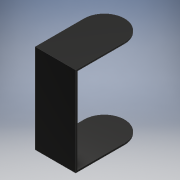
# Autodesk Inventor part: Wrist U-Plate
Saved by Autodesk Inventor 2017 (Build 210142000, 142)
## iProperties
Created: 2018-10-18
Part Number: Wrist U-Plate
Material: Generic
Document SubType Name: Modeling
Designer: Cameron
Density: 1 g/cm^3
Appearance: Glossy - Black
Author: Cameron
Autodesk Inventor part; units mm, degrees
ref_plane "YZ Plane" through (0, 0, 0) normal (1, 0, 0) x (0, 1, 0)
ref_plane "XZ Plane" through (0, 0, 0) normal (0, 1, 0) x (-1, 0, 0)
ref_plane "XY Plane" through (0, 0, 0) normal (0, 0, 1) x (1, 0, 0)
sketch "Sketch1" plane through (0, 0, 0) normal (0, 1, 0) x (-1, 0, 0)
  line L0 (0, 0) -> (24, 0)
  line L1 (24, 0) -> (24, -53)
  line L2 (24, -53) -> (0, -53)
  line L3 (0, -53) -> (0, 0)
  dimension "d0" = 24
  dimension "d1" = 53
  constraints: 8 end point, 2 parallel, 1 horizontal, 1 perpendicular
  measures "d0" distance of L1.end L2.end
  measures "d1" distance of L0.end L1.end
extrude "Extrusion1" add sketch "Sketch1" along normal blind 1
sketch "Sketch2" plane through (0, 1, 0) normal (0, 1, 0) x (1, 0, 0)
  line L0 (-24, 0) -> (0, 0) projected
  line L1 (0, 0) -> (0, 53) projected
  line L2 (-24, 53) -> (-24, 0) projected
  line L3 (-24, 0) -> (0, 0)
  line L4 (0, 0) -> (0, 1)
  line L5 (0, 1) -> (-24, 1)
  line L6 (-24, 1) -> (-24, 0)
  line L7 (0, 53) -> (-24, 53)
  line L8 (-24, 53) -> (-24, 52)
  line L9 (-24, 52) -> (0, 52)
  line L10 (0, 52) -> (0, 53)
  dimension "d4" = 1
  dimension "d5" = 1
  constraints: 16 end point, 4 parallel, 2 horizontal, 2 perpendicular, 2 point on line
  measures "d4" distance of L4.end L3.end
  measures "d5" distance of L8.end L7.end
extrude "Extrusion2" add sketch "Sketch2" along normal blind 40 contours L2 L5 L1 L0 | L2 L7 L1 L9
fillet "Fillet1" radius 12 4 edges at (0, 41, -52.5) (-24, 41, -52.5) (0, 41, -0.5) (-24, 41, -0.5)
body "Solid1"
